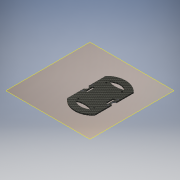
# Autodesk Inventor part: płyta_pod_lipol
Saved by Autodesk Inventor 2017 (Build 210142000, 142)
## iProperties
Created: 2017-05-11
Part Number: płyta_pod_lipol
Material: Ogólny
Document SubType Name: Modeling
Designer: Kuba01
Density: 1 g/cm^3
Appearance: Domyślna
Author: Kuba01
Autodesk Inventor part; units mm, degrees
ref_plane "YZ Plane" through (0, 0, 0) normal (1, 0, 0) x (0, 1, 0)
ref_plane "XZ Plane" through (0, 0, 0) normal (0, 1, 0) x (-1, 0, 0)
ref_plane "XY Plane" through (0, 0, 0) normal (0, 0, 1) x (1, 0, 0)
ref_plane "Płaszczyzna konstrukcyjna1" through (0, 0, 0) normal (0, 0, 1) x (1, 0, 0)
sketch "Szkic1" plane through (0, 0, 0) normal (0, 0, 1) x (1, 0, 0)
  line L0 (-16.5, -47.5) -> (-16.5, 50.5) construction
  line L1 (16.5, -47.5) -> (-16.5, -47.5)
  line L2 (16.5, 50.5) -> (16.5, -47.5) construction
  line L3 (-16.5, 50.5) -> (16.5, 50.5)
  spline S0 degree 3 poles (-35.085094, 0.350302) (-65.123445, -45.85666) (-107.677174, -89.186977) (-160.871239, -134.245964) (-163.540213, -136.506767) (-166.235706, -138.77176) (-168.958028, -141.042) knots 1.00684263 1.00684263 1.00684263 1.00684263 1.95254981 1.95254981 1.95254981 2 2 2 2 construction
  spline S1 degree 3 poles (-168.958035, -141.042006) (-174.842969, -145.949681) (-180.021392, -152.120463) (-183.430993, -158.400223) (-185.92467, -162.993046) (-187.5096, -167.629248) (-187.777285, -172.0593) (-187.941661, -174.779633) (-187.597345, -177.457906) (-186.533873, -179.887417) (-185.566044, -182.098431) (-183.960403, -184.06029) (-181.944828, -185.409391) (-179.841126, -186.817479) (-177.370046, -187.557326) (-174.842104, -187.757319) (-170.645821, -188.089298) (-166.2165, -187.039461) (-161.759498, -185.081578) (-154.903003, -182.06964) (-147.956172, -176.775816) (-142.375954, -170.505914) (-141.930799, -170.005741) (-141.494091, -169.499252) (-141.067481, -168.988346) knots -1.74995257 -1.74995257 -1.74995257 -1.74995257 -1.03595782 -1.03595782 -1.03595782 -0.51376401 -0.51376401 -0.51376401 -0.19310387 -0.19310387 -0.19310387 0.09871784 0.09871784 0.09871784 0.4032988 0.4032988 0.4032988 0.90889088 0.90889088 0.90889088 1.68667586 1.68667586 1.68667586 1.74872267 1.74872267 1.74872267 1.74872267
  spline S2 degree 3 poles (-141.067481, -168.988346) (-116.712468, -140.68912) (-93.293894, -114.867026) (-73.367362, -94.342192) (-61.6586, -82.28187) (-51.151132, -72.048223) (-42.412496, -64.246161) (-37.627468, -59.973975) (-33.366948, -56.428021) (-29.779492, -53.735847) knots 1.1712815 1.1712815 1.1712815 1.1712815 1.58557053 1.58557053 1.58557053 1.82900535 1.82900535 1.82900535 1.96230333 1.96230333 1.96230333 1.96230333
  spline S3 degree 3 poles (-29.779492, -53.735847) (-23.002213, -58.511561) (-16.053637, -61.720133) (-8.95639, -63.196051) (-1.235829, -64.801593) (6.619932, -64.303417) (14.26492, -61.76241) (19.532027, -60.011752) (24.701042, -57.314346) (29.778619, -53.736463) knots 1.04774904 1.04774904 1.04774904 1.04774904 1.36653444 1.36653444 1.36653444 1.71331713 1.71331713 1.71331713 1.95223726 1.95223726 1.95223726 1.95223726
  spline S4 degree 3 poles (29.778619, -53.736463) (34.571432, -57.320947) (40.566429, -62.365096) (47.432495, -68.614281) (65.987099, -85.501849) (90.98262, -111.228833) (117.881656, -141.881406) (125.48107, -150.541255) (133.234406, -159.595591) (141.042009, -168.957931) knots 1.23044004 1.23044004 1.23044004 1.23044004 1.40276207 1.40276207 1.40276207 1.86843878 1.86843878 1.86843878 2 2 2 2
  spline S5 degree 3 poles (141.042009, -168.957931) (145.94969, -174.842884) (152.120487, -180.021325) (158.400263, -183.430935) (162.993086, -185.924612) (167.629288, -187.509541) (172.05934, -187.777227) (174.779673, -187.941603) (177.457946, -187.597287) (179.887458, -186.533815) (182.098472, -185.565985) (184.06033, -183.960345) (185.409431, -181.94477) (186.817519, -179.841068) (187.557366, -177.369988) (187.757359, -174.842045) (188.089339, -170.645763) (187.039501, -166.216442) (185.081618, -161.75944) (182.069681, -154.902945) (176.775856, -147.956114) (170.505954, -142.375896) (169.995852, -141.921904) (169.479183, -141.4767) (168.957931, -141.042009) knots -1.7499544 -1.7499544 -1.7499544 -1.7499544 -1.03595782 -1.03595782 -1.03595782 -0.51376401 -0.51376401 -0.51376401 -0.19310387 -0.19310387 -0.19310387 0.09871784 0.09871784 0.09871784 0.4032988 0.4032988 0.4032988 0.90889088 0.90889088 0.90889088 1.68667586 1.68667586 1.68667586 1.7499544 1.7499544 1.7499544 1.7499544
  spline S6 degree 3 poles (168.957931, -141.042009) (111.993228, -93.537028) (66.637529, -48.185561) (34.855669, -0.000058) knots 1 1 1 1 1.99296801 1.99296801 1.99296801 1.99296801 construction
  spline S7 degree 3 poles (34.855669, -0.000058) (66.637377, 48.185408) (111.993133, 93.536948) (168.957931, 141.042009) knots 1.00703033 1.00703033 1.00703033 1.00703033 2 2 2 2 construction
  spline S8 degree 3 poles (168.957931, 141.042009) (174.842884, 145.94969) (180.021325, 152.120487) (183.430935, 158.400263) (185.924612, 162.993086) (187.509541, 167.629288) (187.777227, 172.05934) (187.941603, 174.779673) (187.597287, 177.457946) (186.533815, 179.887458) (185.565985, 182.098472) (183.960345, 184.06033) (181.94477, 185.409431) (179.841068, 186.817519) (177.369988, 187.557366) (174.842045, 187.757359) (170.645763, 188.089339) (166.216442, 187.039501) (161.75944, 185.081618) (154.902945, 182.069681) (147.956114, 176.775856) (142.375896, 170.505954) (141.93073, 170.005769) (141.494012, 169.499268) (141.067392, 168.98835) knots -1.7499544 -1.7499544 -1.7499544 -1.7499544 -1.03595782 -1.03595782 -1.03595782 -0.51376401 -0.51376401 -0.51376401 -0.19310387 -0.19310387 -0.19310387 0.09871784 0.09871784 0.09871784 0.4032988 0.4032988 0.4032988 0.90889088 0.90889088 0.90889088 1.68667586 1.68667586 1.68667586 1.74872416 1.74872416 1.74872416 1.74872416 construction
  spline S9 degree 3 poles (141.067392, 168.98835) (116.712447, 140.689096) (93.29391, 114.86699) (73.367396, 94.342151) (61.658634, 82.281814) (51.151162, 72.048159) (42.412523, 64.246094) (37.627506, 59.973916) (33.366993, 56.427969) (29.779541, 53.7358) knots 1.17128149 1.17128149 1.17128149 1.17128149 1.58557053 1.58557053 1.58557053 1.82900558 1.82900558 1.82900558 1.96230334 1.96230334 1.96230334 1.96230334 construction
  spline S10 degree 3 poles (29.779541, 53.7358) (23.00225, 58.511525) (16.053664, 61.720107) (8.956408, 63.196032) (1.235842, 64.80158) (-6.619923, 64.30341) (-14.264913, 61.762407) (-19.532023, 60.011751) (-24.70104, 57.314346) (-29.778619, 53.736463) knots 1.04774897 1.04774897 1.04774897 1.04774897 1.36653452 1.36653452 1.36653452 1.71331713 1.71331713 1.71331713 1.95223726 1.95223726 1.95223726 1.95223726
  spline S11 degree 3 poles (-29.778619, 53.736463) (-34.571432, 57.320947) (-40.566429, 62.365096) (-47.432495, 68.614281) (-65.987099, 85.501849) (-90.98262, 111.228833) (-117.881656, 141.881406) (-125.48107, 150.541255) (-133.234406, 159.595591) (-141.042009, 168.957931) knots 1.23044004 1.23044004 1.23044004 1.23044004 1.40276207 1.40276207 1.40276207 1.86843878 1.86843878 1.86843878 2 2 2 2 construction
  spline S12 degree 3 poles (-141.042009, 168.957931) (-145.94969, 174.842884) (-152.120487, 180.021325) (-158.400263, 183.430935) (-162.993086, 185.924612) (-167.629288, 187.509541) (-172.05934, 187.777227) (-174.779673, 187.941603) (-177.457946, 187.597287) (-179.887458, 186.533815) (-182.098472, 185.565985) (-184.06033, 183.960345) (-185.409431, 181.94477) (-186.817519, 179.841068) (-187.557366, 177.369988) (-187.757359, 174.842045) (-188.089339, 170.645763) (-187.039501, 166.216442) (-185.081618, 161.75944) (-182.069681, 154.902945) (-176.775856, 147.956114) (-170.505954, 142.375896) (-169.995852, 141.921904) (-169.479183, 141.4767) (-168.957931, 141.042009) knots -1.7499544 -1.7499544 -1.7499544 -1.7499544 -1.03595782 -1.03595782 -1.03595782 -0.51376401 -0.51376401 -0.51376401 -0.19310387 -0.19310387 -0.19310387 0.09871784 0.09871784 0.09871784 0.4032988 0.4032988 0.4032988 0.90889088 0.90889088 0.90889088 1.68667586 1.68667586 1.68667586 1.7499544 1.7499544 1.7499544 1.7499544
  spline S13 degree 3 poles (-168.957931, 141.042009) (-111.993306, 93.537093) (-66.634651, 48.181164) (-35.085094, 0.350302) knots 1 1 1 1 1.99296665 1.99296665 1.99296665 1.99296665 construction
  spline S14 degree 3 poles (15.08474, 32.081826) (13.142615, 27.920021) (11.206834, 23.755267) (7.347081, 15.418016) (5.423125, 11.245533) (3.50551, 7.070128) knots 0 0 0 0 1.37779618 1.37779618 2.75620579 2.75620579 2.75620579 2.75620579 construction
  arc A0 (3.50551, 7.070128) -> (-3.550162, 7.111441) centre (-0.064535, -0.117868) ccw
  spline S15 degree 3 poles (-3.550162, 7.111441) (-5.476159, 11.293082) (-7.408923, 15.471593) (-11.287085, 23.820373) (-13.232467, 27.990624) (-15.184617, 32.157717) knots 0 0 0 0 1.38115979 1.38115979 2.76166682 2.76166682 2.76166682 2.76166682 construction
  spline S16 degree 3 poles (-15.184617, 32.157717) (-14.754715, 32.524347) (-14.315487, 32.879522) (-13.401907, 33.58056) (-12.927392, 33.92514) (-12.444135, 34.257559) knots 0 0 0 0 0.49064646 0.49064646 1 1 1 1
  spline S17 degree 3 poles (-12.444135, 34.257559) (-9.857516, 31.263166) (-7.370332, 28.095019) (-3.226905, 21.915373) (-1.464317, 18.86972) (-0.029639, 15.697104) knots 0 0 0 0 1.18706736 1.18706736 2.2295227 2.2295227 2.2295227 2.2295227
  spline S18 degree 3 poles (-0.029639, 15.697104) (1.394779, 18.864276) (3.146428, 21.904712) (7.267313, 28.073431) (9.741557, 31.234617) (12.316482, 34.222704) knots 0 0 0 0 1.04182291 1.04182291 2.22753004 2.22753004 2.22753004 2.22753004
  spline S19 degree 3 poles (12.316482, 34.222704) (12.805198, 33.884055) (13.28481, 33.532857) (14.207654, 32.81808) (14.651041, 32.455846) (15.08474, 32.081826) knots 0 0 0 0 0.50937249 0.50937249 1 1 1 1
  spline S20 degree 3 poles (-19.948357, 42.291714) (-14.639949, 45.838264) (-9.990985, 47.660697) (-2.091787, 49.301941) (1.677222, 49.331262) (9.761575, 47.76592) (14.518581, 45.908732) (19.884685, 42.334177) knots 0 0 0 0 1.91524131 1.91524131 3.69438874 3.69438874 5.68840016 5.68840016 5.68840016 5.68840016 construction
  spline S21 degree 3 poles (19.884685, 42.334177) (13.583668, 39.654933) (6.996486, 38.105537) (-3.242366, 38.040322) (-6.597665, 38.388751) (-13.364764, 39.812974) (-16.709843, 40.903142) (-19.948357, 42.291714) knots 0 0 0 0 2.05409443 2.05409443 3.07151826 3.07151826 4.128565 4.128565 4.128565 4.128565
  circle A1 centre (-173.423564, 173.187828) radius 3
  circle A2 centre (173.294495, -173.423564) radius 3
  circle A3 centre (173.241161, 173.241161) radius 3
  circle A4 centre (-173.370231, -173.476898) radius 3
  spline S22 degree 3 poles (-19.066093, -42.869125) (-12.882074, -40.751924) (-6.517551, -39.59928) (6.547635, -39.59651) (12.903023, -40.74369) (19.078711, -42.861037) knots 0 0 0 0 1.96092247 1.96092247 3.91949067 3.91949067 3.91949067 3.91949067 construction
  spline S23 degree 3 poles (19.078711, -42.861037) (14.864666, -45.563042) (10.225957, -47.709734) (1.45827, -49.346262) (-2.32179, -49.284891) (-9.747617, -47.680221) (-14.038512, -46.090792) (-19.066093, -42.869125) knots 0 0 0 0 1.5017693 1.5017693 2.66720704 2.66720704 3.77054668 3.77054668 3.77054668 3.77054668
  spline S24 degree 3 poles (-14.516561, -32.673383) (-12.636802, -28.474571) (-10.750685, -24.278615) (-6.966619, -15.894413) (-5.068682, -11.706181) (-3.164387, -7.520833) knots 0 0 0 0 1.38011477 1.38011477 2.75957612 2.75957612 2.75957612 2.75957612 construction
  arc A5 (-3.164387, -7.520833) -> (3.168342, -7.463715) centre (-0.064535, -0.117868) ccw
  spline S25 degree 3 poles (3.168342, -7.463715) (5.085541, -11.667908) (6.995965, -15.875184) (10.800733, -24.290442) (12.69509, -28.498407) (14.582623, -32.709436) knots 0 0 0 0 1.38621048 1.38621048 2.77062343 2.77062343 2.77062343 2.77062343 construction
  spline S26 degree 3 poles (14.582623, -32.709436) (14.13991, -33.096217) (13.662069, -33.486083) (12.716313, -34.222379) (12.21496, -34.593642) (11.712763, -34.945387) knots 0 0 0 0 0.49185835 0.49185835 1 1 1 1
  spline S27 degree 3 poles (11.712763, -34.945387) (9.276978, -32.103289) (6.942538, -29.102251) (3.034739, -23.232824) (1.370156, -20.340004) (0.003694, -17.328259) knots 0 0 0 0 1.12292095 1.12292095 2.11343337 2.11343337 2.11343337 2.11343337 construction
  spline S28 degree 3 poles (0.003694, -17.328259) (-1.356274, -20.333171) (-3.013893, -23.219487) (-6.906842, -29.076217) (-9.233125, -32.070858) (-11.66075, -34.906916) knots 0 0 0 0 0.98950049 0.98950049 2.1113335 2.1113335 2.1113335 2.1113335
  spline S29 degree 3 poles (-11.66075, -34.906916) (-12.164863, -34.554062) (-12.659287, -34.188046) (-13.611319, -33.442296) (-14.069007, -33.063947) (-14.516561, -32.673383) knots 0 0 0 0 0.50881737 0.50881737 1 1 1 1
  line L4 (-35.085094, 0.350302) -> (-35.085094, 49.099838)
  line L5 (-35.085094, 0.350302) -> (-35.085094, -48.281474)
  line L6 (34.855669, -0.000058) -> (34.855669, -48.547874)
  line L7 (34.855669, -0.000058) -> (34.855669, 49.277496)
  arc A6 (34.855669, 49.277496) -> (-35.085094, 49.099838) centre (-0.029639, 15.697104) ccw
  arc A7 (-35.085094, -48.281474) -> (34.855669, -48.547874) centre (0.003694, -17.328259) ccw
  circle A8 centre (-20, -35) radius 2
  line L8 (-277.818739, 0) -> (277.818714, 0)
  line L9 (0, -277.778257) -> (0, 277.778257)
  circle A9 centre (20, -35) radius 2
  circle A10 centre (-20, 35) radius 2
  circle A11 centre (20, 35) radius 2
  arc A12 (28.355669, 7.5) -> (23.355669, 7.5) centre (25.855669, 7.5) ccw
  arc A13 (23.355669, -7.5) -> (28.355669, -7.5) centre (25.855669, -7.5) ccw
  line L10 (28.355669, -7.5) -> (28.355669, 7.5)
  line L11 (23.355669, 7.5) -> (23.355669, -7.5)
  arc A14 (-23.355669, 7.5) -> (-28.355669, 7.5) centre (-25.855669, 7.5) ccw
  arc A15 (-28.355669, -7.5) -> (-23.355669, -7.5) centre (-25.855669, -7.5) ccw
  line L12 (-28.355669, -7.5) -> (-28.355669, 7.5)
  line L13 (-23.355669, 7.5) -> (-23.355669, -7.5)
  line L14 (19.884685, 42.334177) -> (5.5616, 51.719428) construction
  line L15 (5.5616, 51.719428) -> (-5.507512, 51.719428) construction
  line L16 (-5.507512, 51.719428) -> (-19.948357, 42.291714) construction
  spline S30 degree 3 poles (19.884685, 42.334177) (5.5616, 51.719428) (-5.507512, 51.719428) (-19.948357, 42.291714) knots 1 1 1 1 2 2 2 2
  line L17 (19.884685, 42.334177) -> (6.838806, 36.499399) construction
  line L18 (6.838806, 36.499399) -> (-7.484612, 36.499399) construction
  line L19 (-7.484612, 36.499399) -> (-19.948357, 42.291714) construction
  spline S31 degree 3 poles (19.884685, 42.334177) (6.838806, 36.499399) (-7.484612, 36.499399) (-19.948357, 42.291714) knots 1 1 1 1 2 2 2 2
  spline S32 degree 3 poles (-19.948357, -42.291714) (-18.746641, -43.094581) (-16.376096, -44.544624) (-13.501106, -45.983476) (-10.692066, -47.156791) (-8.496008, -47.889736) (-5.805048, -48.565032) (-3.689231, -48.918937) (-1.070138, -49.1397) (1.014806, -49.141741) (3.633449, -48.926153) (5.748573, -48.576507) (8.438356, -47.906787) (10.633281, -47.178527) (13.440795, -46.011363) (16.314211, -44.578944) (18.683547, -43.134298) (19.884685, -42.334177) knots 1.0724773 1.0724773 1.0724773 1.0724773 1.1438362 1.2151951 1.25087454 1.32223344 1.35791289 1.42927178 1.46495123 1.53631013 1.57198957 1.64334847 1.67902792 1.75038681 1.78606626 1.85742515 1.92878405 1.92878405 1.92878405 1.92878405
  line L20 (19.884685, -42.334177) -> (6.838806, -36.499399) construction
  line L21 (6.838806, -36.499399) -> (-7.484612, -36.499399) construction
  line L22 (-7.484612, -36.499399) -> (-19.948357, -42.291714) construction
  spline S33 degree 3 poles (19.884685, -42.334177) (6.838806, -36.499399) (-7.484612, -36.499399) (-19.948357, -42.291714) knots 1 1 1 1 2 2 2 2
  point P0 (0, 0)
  dimension "d0" = 4
  dimension "d3" = 3.5
  dimension "d4" = 12.5
  dimension "d5" = 5
  dimension "d6" = 9
  dimension "d7" = 7.5
  constraints: 16 end point, 14 symmetric about line, 12 point on circle, 10 centre point, 2 coincident, 2 point on line, 2 vertical, 1 horizontal, 1 parallel, 1 tangent, 15 other
  measures "d0" diameter of A8
  measures "d3" distance from line of A8.centre L0
  measures "d4" distance from line of A8.centre L1
  measures "d5" diameter of A12
  measures "d6" distance from line of L7 A12.centre
  measures "d7" distance from line of L8 A12.centre
sketch "Szkic1 outline for Wyciągnięcie proste1" plane through (0, 0, 0) normal (0, 0, 1) x (1, 0, 0)
  line L0 (-35.085094, 0.350302) -> (-35.085094, 49.099838)
  line L1 (-35.085094, -48.281474) -> (-35.085094, 0.350302)
  arc A0 (-35.085094, 49.099838) -> (34.855669, 49.277496) centre (-0.029639, 15.697104) cw
  arc A1 (34.855669, -48.547874) -> (-35.085094, -48.281474) centre (0.003694, -17.328259) cw
  line L2 (34.855669, 49.277496) -> (34.855669, -0.000058)
  line L3 (34.855669, -0.000058) -> (34.855669, -48.547874)
  circle A2 centre (-20, -35) radius 2
  spline S0 degree 3 poles (19.884685, -42.334177) (6.838806, -36.499399) (-7.484612, -36.499399) (-19.948357, -42.291714) knots 0 0 0 0 1 1 1 1
  spline S1 degree 3 poles (-19.948357, -42.291714) (-18.746641, -43.094581) (-16.376096, -44.544624) (-13.501106, -45.983476) (-10.692066, -47.156791) (-8.496008, -47.889736) (-5.805048, -48.565032) (-3.689231, -48.918937) (-1.070138, -49.1397) (1.014806, -49.141741) (3.633449, -48.926153) (5.748573, -48.576507) (8.438356, -47.906787) (10.633281, -47.178527) (13.440795, -46.011363) (16.314211, -44.578944) (18.683547, -43.134298) (19.884685, -42.334177) knots 0 0 0 0 0.08333333 0.16666667 0.20833333 0.29166667 0.33333333 0.41666667 0.45833333 0.54166667 0.58333333 0.66666667 0.70833333 0.79166667 0.83333333 0.91666667 1 1 1 1
  line L4 (-28.355669, 7.5) -> (-28.355669, -7.5)
  arc A3 (-28.355669, -7.5) -> (-23.355669, -7.5) centre (-25.855669, -7.5) ccw
  line L5 (-23.355669, -7.5) -> (-23.355669, 7.5)
  arc A4 (-23.355669, 7.5) -> (-28.355669, 7.5) centre (-25.855669, 7.5) ccw
  circle A5 centre (20, -35) radius 2
  line L6 (28.355669, 7.5) -> (28.355669, -7.5)
  arc A6 (23.355669, 7.5) -> (28.355669, 7.5) centre (25.855669, 7.5) cw
  line L7 (23.355669, -7.5) -> (23.355669, 7.5)
  arc A7 (28.355669, -7.5) -> (23.355669, -7.5) centre (25.855669, -7.5) cw
  circle A8 centre (-20, 35) radius 2
  spline S2 degree 3 poles (19.884685, 42.334177) (5.5616, 51.719428) (-5.507512, 51.719428) (-19.948357, 42.291714) knots 0 0 0 0 1 1 1 1
  spline S3 degree 3 poles (19.884685, 42.334177) (6.838806, 36.499399) (-7.484612, 36.499399) (-19.948357, 42.291714) knots 0 0 0 0 1 1 1 1
  circle A9 centre (20, 35) radius 2
extrude "Wyciągnięcie proste1" add sketch "Szkic1 outline for Wyciągnięcie proste1" along normal blind 3
sketch "Szkic2" plane through (0, 0, 0) normal (0, 0, -1) x (-1, 0, 0)
  ellipse E0 centre (-36.5599, 0) end of major axis (-43.081778, 0) minor radius 6
  circle A0 centre (-32.044255, 12.339629) radius 2
  circle A1 centre (-32.044255, -12.339629) radius 2
  ellipse E1 centre (36.5599, 0) end of major axis (43.081778, 0) minor radius 6
  circle A2 centre (32.044255, 12.339629) radius 2
  circle A3 centre (32.044255, -12.339629) radius 2
  point P0 (0, 0)
  constraints: 4 centre point, 14 other
extrude "Wyciągnięcie proste2" cut sketch "Szkic2" against normal through all
sketch "Szkic3" plane through (0, 0, 0) normal (0, 0, -1) x (-1, 0, 0)
  circle A0 centre (-29.855669, -45.12143) radius 1.5
  circle A1 centre (-29.855669, 45.469872) radius 1.5
  circle A2 centre (30.010159, 45.469872) radius 1.5
  circle A3 centre (30.010159, -45.12143) radius 1.5
  point P0 (0, 0)
  constraints: 4 centre point, 8 other
extrude "Wyciągnięcie proste3" cut sketch "Szkic3" against normal through all
